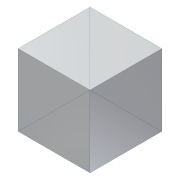
# Autodesk Inventor part: Extrude
Saved by Autodesk Inventor 2014 (Build 180170000, 170)
## iProperties
Created: 2014-01-15
Part Number: Extrude
Material: Generic
Document SubType Name: Modeling
Designer: Yogesh
Density: 1 g/cm^3
Appearance: Clear
Author: Yogesh
Autodesk Inventor part; units mm, degrees
ref_plane "YZ Plane" through (0, 0, 0) normal (1, 0, 0) x (0, 1, 0)
ref_plane "XZ Plane" through (0, 0, 0) normal (0, 1, 0) x (-1, 0, 0)
sketch "Sketch1" plane through (0, 0, 0) normal (0, 0, 1) x (1, 0, 0)
  line L0 (50, 50) -> (50, 0)
  line L1 (-50, -50) -> (50, -50)
  line L2 (50, -50) -> (50, 50)
  line L3 (50, 50) -> (-50, 50)
  line L4 (-50, 50) -> (-50, -50)
  line L5 (-50, -50) -> (50, 50) construction
  line L6 (50, -50) -> (-50, 50) construction
  point P0 (0, 0)
  constraints: 14 end point, 2 midpoint, 2 parallel, 1 horizontal, 1 perpendicular
ref_plane "Work Plane1" through (0, 0, -100) normal (0, 0, 1) x (1, 0, 0)
extrude "Extrusion2" add sketch "Sketch1" against normal blind 100
body "Solid3"
